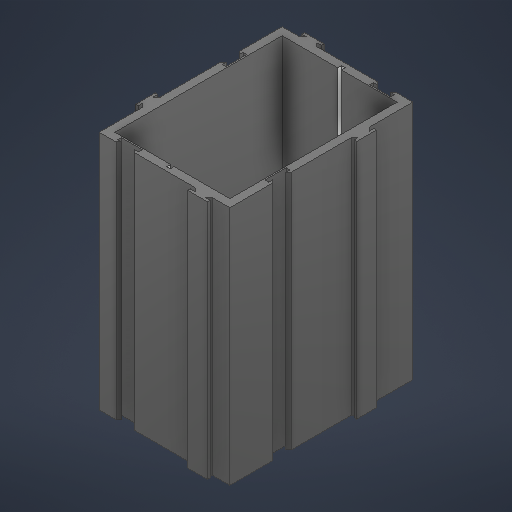
# Autodesk Inventor part: box
Saved by Autodesk Inventor 2027 (Build 310192060, 192F)
## iProperties
Created: 2026-06-08
Part Number: box
Material: Ogólny
Document SubType Name: Modeling
Designer: User
Density: 1 g/cm^3
Appearance: Domyślna
Author: User
Autodesk Inventor part; units mm, degrees
ref_plane "YZ Plane" through (0, 0, 0) normal (1, 0, 0) x (0, 1, 0)
ref_plane "XZ Plane" through (0, 0, 0) normal (0, 1, 0) x (-1, 0, 0)
ref_plane "XY Plane" through (0, 0, 0) normal (0, 0, 1) x (1, 0, 0)
sketch "Szkic1" plane through (0, 0, 0) normal (0, 1, 0) x (-1, 0, 0)
  line L0 (-25, -35) -> (25, -35)
  line L1 (25, -35) -> (25, 35)
  line L2 (25, 35) -> (-25, 35)
  line L3 (-25, 35) -> (-25, -35)
  line L4 (-25, -35) -> (25, 35) construction
  line L5 (25, -35) -> (-25, 35) construction
  line L6 (-22, -32) -> (22, -32)
  line L7 (22, -32) -> (22, 32)
  line L8 (22, 32) -> (-22, 32)
  line L9 (-22, 32) -> (-22, -32)
  line L10 (-22, -32) -> (22, 32) construction
  line L11 (22, -32) -> (-22, 32) construction
  line L12 (25, 35) -> (18.5607, 35)
  line L13 (25, 35) -> (31.4393, 35) construction
  line L14 (18.5607, 35) -> (17.5, 33.9393)
  line L15 (17.5, 33.9393) -> (19, 33.9393)
  line L16 (19, 33.9393) -> (19, 32.5393)
  line L17 (-25, 35) -> (-23, 35) construction
  line L18 (0, 32) -> (0, 35) construction
  line L19 (18.5607, 35) -> (32.6482, 35) construction
  line L20 (11.4393, 35) -> (29.6482, 35) construction
  line L21 (19, 32.5393) -> (15, 32.5393)
  line L22 (15, 32.5393) -> (15, 35) construction
  line L23 (11.4393, 35) -> (12.5, 33.9393)
  line L24 (12.5, 33.9393) -> (11, 33.9393)
  line L25 (11, 33.9393) -> (11, 32.5393)
  line L26 (11, 32.5393) -> (15, 32.5393)
  line L27 (-18.5607, 35) -> (-17.5, 33.9393) construction
  line L28 (-17.5, 33.9393) -> (-19, 33.9393) construction
  line L29 (-19, 32.5393) -> (-15, 32.5393) construction
  line L30 (-15, 32.5393) -> (-15, 35) construction
  line L31 (-11.4393, 35) -> (-12.5, 33.9393) construction
  line L32 (-11, 32.5393) -> (-15, 32.5393) construction
  line L33 (-11, 33.9393) -> (-11, 32.5393) construction
  line L34 (-12.5, 33.9393) -> (-11, 33.9393) construction
  line L35 (-19, 33.9393) -> (-19, 32.5393) construction
  line L36 (22, 0) -> (-22, 0) construction
  line L37 (25, 0) -> (22, 0) construction
  line L38 (18.5607, -35) -> (17.5, -33.9393) construction
  line L39 (17.5, -33.9393) -> (19, -33.9393) construction
  line L40 (19, -33.9393) -> (19, -32.5393) construction
  line L41 (19, -32.5393) -> (15, -32.5393) construction
  line L42 (15, -32.5393) -> (15, -35) construction
  line L43 (11.4393, -35) -> (12.5, -33.9393) construction
  line L44 (11, -32.5393) -> (15, -32.5393) construction
  line L45 (11, -33.9393) -> (11, -32.5393) construction
  line L46 (12.5, -33.9393) -> (11, -33.9393) construction
  line L47 (-11.4393, -35) -> (-12.5, -33.9393)
  line L48 (-12.5, -33.9393) -> (-11, -33.9393)
  line L49 (-15, -32.5393) -> (-15, -35) construction
  line L50 (-11, -32.5393) -> (-15, -32.5393)
  line L51 (-18.5607, -35) -> (-17.5, -33.9393)
  line L52 (-17.5, -33.9393) -> (-19, -33.9393)
  line L53 (-19, -32.5393) -> (-15, -32.5393)
  line L54 (-11, -33.9393) -> (-11, -32.5393)
  line L55 (-19, -33.9393) -> (-19, -32.5393)
  line L56 (25, 11.4393) -> (23.9393, 12.5) construction
  line L57 (23.9393, 12.5) -> (23.9393, 11) construction
  line L58 (23.9393, 11) -> (22.5393, 11) construction
  line L59 (22.5393, 11) -> (22.5393, 15) construction
  line L60 (22.5393, 15) -> (24.8, 15) construction
  line L61 (25, 18.5607) -> (23.9393, 17.5) construction
  line L62 (22.5393, 19) -> (22.5393, 15) construction
  line L63 (23.9393, 19) -> (22.5393, 19) construction
  line L64 (23.9393, 17.5) -> (23.9393, 19) construction
  line L65 (25, -11.4393) -> (23.9393, -12.5)
  line L66 (23.9393, -12.5) -> (23.9393, -11)
  line L67 (23.9393, -11) -> (22.5393, -11)
  line L68 (22.5393, -11) -> (22.5393, -15)
  line L69 (25, -18.5607) -> (23.9393, -17.5)
  line L70 (23.9393, -17.5) -> (23.9393, -19)
  line L71 (22.5393, -15) -> (24.8, -15) construction
  line L72 (22.5393, -19) -> (22.5393, -15)
  line L73 (23.9393, -19) -> (22.5393, -19)
  line L74 (-25, 11.4393) -> (-23.9393, 12.5)
  line L75 (-23.9393, 12.5) -> (-23.9393, 11)
  line L76 (-23.9393, 11) -> (-22.5393, 11)
  line L77 (-22.5393, 11) -> (-22.5393, 15)
  line L78 (-25, 18.5607) -> (-23.9393, 17.5)
  line L79 (-23.9393, 17.5) -> (-23.9393, 19)
  line L80 (-22.5393, 15) -> (-24.8, 15) construction
  line L81 (-22.5393, 19) -> (-22.5393, 15)
  line L82 (-23.9393, 19) -> (-22.5393, 19)
  line L83 (-25, -11.4393) -> (-23.9393, -12.5) construction
  line L84 (-23.9393, -12.5) -> (-23.9393, -11) construction
  line L85 (-23.9393, -11) -> (-22.5393, -11) construction
  line L86 (-22.5393, -11) -> (-22.5393, -15) construction
  line L87 (-22.5393, -15) -> (-24.8, -15) construction
  line L88 (-25, -18.5607) -> (-23.9393, -17.5) construction
  line L89 (-22.5393, -19) -> (-22.5393, -15) construction
  line L90 (-23.9393, -17.5) -> (-23.9393, -19) construction
  line L91 (-23.9393, -19) -> (-22.5393, -19) construction
  line L92 (-11.4393, 35) -> (-12.5, 36.0607)
  line L93 (-12.5, 36.0607) -> (-11, 36.0607)
  line L94 (-15, 37.4607) -> (-15, 35)
  line L95 (-11, 37.4607) -> (-15, 37.4607)
  line L96 (-18.5607, 35) -> (-17.5, 36.0607)
  line L97 (-17.5, 36.0607) -> (-19, 36.0607)
  line L98 (-19, 37.4607) -> (-15, 37.4607)
  line L99 (-11, 36.0607) -> (-11, 37.4607)
  line L100 (-19, 36.0607) -> (-19, 37.4607)
  line L101 (18.5607, -35) -> (17.5, -36.0607)
  line L102 (17.5, -36.0607) -> (19, -36.0607)
  line L103 (19, -36.0607) -> (19, -37.4607)
  line L104 (19, -37.4607) -> (15, -37.4607)
  line L105 (11, -37.4607) -> (15, -37.4607)
  line L106 (15, -37.4607) -> (15, -35) construction
  line L107 (11.4393, -35) -> (12.5, -36.0607)
  line L108 (11, -36.0607) -> (11, -37.4607)
  line L109 (12.5, -36.0607) -> (11, -36.0607)
  line L110 (25, 11.4393) -> (26.0607, 12.5)
  line L111 (26.0607, 12.5) -> (26.0607, 11)
  line L112 (26.0607, 11) -> (27.4607, 11)
  line L113 (27.4607, 11) -> (27.4607, 15)
  line L114 (25, 18.5607) -> (26.0607, 17.5)
  line L115 (26.0607, 17.5) -> (26.0607, 19)
  line L116 (27.4607, 15) -> (25.2, 15) construction
  line L117 (27.4607, 19) -> (27.4607, 15)
  line L118 (26.0607, 19) -> (27.4607, 19)
  line L119 (-26.0607, -19) -> (-27.4607, -19)
  line L120 (-26.0607, -17.5) -> (-26.0607, -19)
  line L121 (-25, -18.5607) -> (-26.0607, -17.5)
  line L122 (-27.4607, -11) -> (-27.4607, -15)
  line L123 (-27.4607, -15) -> (-25.2, -15) construction
  line L124 (-26.0607, -11) -> (-27.4607, -11)
  line L125 (-26.0607, -12.5) -> (-26.0607, -11)
  line L126 (-25, -11.4393) -> (-26.0607, -12.5)
  line L127 (-27.4607, -19) -> (-27.4607, -15)
  point P0 (0, 0)
  point P1 (-11.4393, 35)
  point P2 (-18.5607, 35)
  point P3 (-18.5607, -35)
  point P4 (-11.4393, -35)
  point P5 (11.4393, -35)
  point P6 (18.5607, 35)
  point P7 (0, 33.5)
  point P8 (15, 33.7697)
  point P9 (23.5, 0)
  point P10 (-15, 33.7697)
  point P11 (23.6697, 15)
  point P12 (23.6697, -15)
  point P13 (-23.6697, 15)
  point P14 (-23.6697, -15)
  point P15 (23.6697, -15)
  point P16 (-25, 18.5607)
  point P17 (-25, 11.4393)
  point P18 (-25, -18.5607)
  point P19 (25, -18.5607)
  point P20 (25, -11.4393)
  point P21 (-15, 36.2303)
  point P22 (26.3303, 15)
  point P23 (-26.3303, -15)
  point P24 (-25, -18.5607)
  point P25 (18.5607, -35)
  point P26 (11.4393, -35)
  point P27 (-18.5607, 35)
  point P28 (-11.4393, 35)
  dimension "d0" = 50
  dimension "d1" = 70
  dimension "d2" = 44
  dimension "d3" = 64
  dimension "d6" = 1.5
  dimension "d7" = 135
  dimension "d8" = 1.5
  dimension "d9" = 1.4
  dimension "d15" = 2
  dimension "d23" = 4
  dimension "d29" = 45
  dimension "d34" = 1.5
  dimension "d35" = 1.5
  dimension "d36" = 1.4
  dimension "d37" = 4
  dimension "d38" = 45
  dimension "d76" = 1.1303
  dimension "d90" = 20
  dimension "d91" = 10
  constraints: 256 end point, 102 symmetric about line, 15 midpoint, 10 parallel, 7 point on line, 4 horizontal, 4 perpendicular, 2 collinear, 2 vertical
  measures "d0" distance of L2.end L1.end
  measures "d1" distance of L1.end L0.end
  measures "d2" distance of L8.end L7.end
  measures "d3" distance of L7.end L6.end
  measures "d6" distance of L12.end L14.end
  measures "d7" angle of L14 L12
  measures "d8" distance of L14.end L15.end
  measures "d9" distance of L15.end L16.end
  measures "d15" distance of L2.end L17.end
  measures "d23" distance of L16.end L21.end
  measures "d29" angle of L24 L23
  measures "d34" distance of L56.start L56.end
  measures "d35" distance of L56.end L57.end
  measures "d36" distance of L57.end L58.end
  measures "d37" distance of L58.end L59.end
  measures "d38" angle of L64 L61
  measures "d76" distance of L68.end point (23.67, -15)
  measures "d90" distance from line of L2 point (23.67, 15)
  measures "d91" distance from line of L1 point (15, 33.77)
extrude "Wyciągnięcie proste1" add sketch "Szkic1" along normal blind 90 contours L3 L74 L75 L76 L77 L81 L82 L79 L78 L2 L23 L24 L25 L26 L21 L16 L15 L14 L1 L65 L66 L67 L68 L72 L73 L70 L69 L0 L47 L48 L54 L50 L53 L55 L52 L51 | L121 L120 L119 L127 L122 L124 L125 L126 L3 | L0 L101 L102 L103 L104 L105 L108 L109 L107 | L96 L97 L100 L98 L94 L2 | L94 L95 L99 L93 L92 L2 | L1 L114 L115 L118 L117 L113 L112 L111 L110
extrude "Wyciągnięcie proste2" add sketch "Szkic1" against normal blind 2 contours L3 L74 L75 L76 L77 L81 L82 L79 L78 L2 L23 L24 L25 L26 L21 L16 L15 L14 L1 L65 L66 L67 L68 L72 L73 L70 L69 L0 L47 L48 L54 L50 L53 L55 L52 L51 | L121 L120 L119 L127 L122 L124 L125 L126 L3 | L0 L101 L102 L103 L104 L105 L108 L109 L107 | L96 L97 L100 L98 L94 L2 | L94 L95 L99 L93 L92 L2 | L1 L114 L115 L118 L117 L113 L112 L111 L110 | L9 L8 L7 L6
offset faces "Rozmiar1" outward -0.2 faces at (-19, 28.6667, -36.994) (-17.8536, 28.6667, -35.7071) (-13.6667, 28.6667, -37.4607) (-11, 28.6667, -36.5273) (-11.7929, 28.6667, -35.3536) (-12, 28.6667, -36.0607) (-18.5, 28.6667, -36.0607) (-26.0607, 28.6667, 12) (-26.5273, 28.6667, 11) (-25.7071, 28.6667, 17.8536) (-26.994, 28.6667, 19) (-26.0607, 28.6667, 18.5) (-25.3536, 28.6667, 11.7929) (-27.4607, 28.6667, 13.6667) (16.3333, 59.3333, 37.4607) (19, 59.3333, 36.5273) (18.2071, 59.3333, 35.3536) (18, 59.3333, 36.0607) (11.5, 59.3333, 36.0607) (11, 59.3333, 36.994) (12.1464, 59.3333, 35.7071) (26.0607, 59.3333, -11.5) (26.994, 59.3333, -11) (27.4607, 59.3333, -16.3333) (26.5273, 59.3333, -19) (26.0607, 59.3333, -18)
move faces "Przesuń1" translate (0.05, 0, 0) faces at (26.2607, 59.3333, -17.8) (26.2607, 59.3333, -11.7) (27.2607, 59.3333, -16.2667)
move faces "Przesuń2" translate (-0.05, 0, 0) faces at (-26.2607, 59.3333, 17.6114) (-26.2607, 59.3333, 11.7943) (-27.2607, 59.3333, 16.2667)
move faces "Przesuń3" translate (0, 0, -0.05) faces at (-11.7943, 59.3333, -36.2607) (-17.6114, 59.3333, -36.2607) (-16.2667, 59.3333, -37.2607)
move faces "Przesuń4" translate (0, 0, 0.05) faces at (13.7333, 28.6667, 37.2607) (18.2057, 28.6667, 36.2607) (12.3886, 28.6667, 36.2607)
sketch "Szkic2" plane through (0, 90, 0) normal (0, 1, 0) x (1, 0, 0)
  line L0 (-0.7, -33.5) -> (0.7, -33.5)
  line L1 (0.7, -33.5) -> (0.7, 33.5)
  line L2 (0.7, 33.5) -> (-0.7, 33.5)
  line L3 (-0.7, 33.5) -> (-0.7, -33.5)
  line L4 (-0.7, -33.5) -> (0.7, 33.5) construction
  line L5 (0.7, -33.5) -> (-0.7, 33.5) construction
  point P0 (0, 0)
  dimension "d92" = 1.4
  dimension "d93" = 67
  constraints: 12 end point, 2 midpoint, 2 parallel, 1 horizontal, 1 perpendicular
  measures "d92" distance of L2.end L1.end
  measures "d93" distance of L1.end L0.end
extrude "Wyciągnięcie proste3" cut sketch "Szkic2" against normal up to surface (90 mm away)
equation "\"Offcenter\" = 15"
